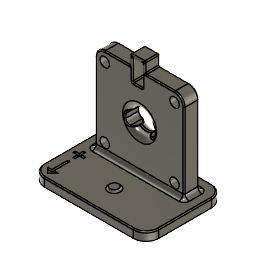
SOC Monitor Assembly (Autodesk Fusion 360 archive; units mm, degrees)
design "Mount"
part number: 2026-03-20-00-19-52-846
Autodesk Fusion 360 part; units mm, degrees
sketch "Base Bottom" plane through (0, 0, 0) normal (0, 0, 1) x (1, 0, 0)
  line L0 (-21, -18.5) -> (21, -18.5)
  line L1 (27, -12.5) -> (27, 12.5)
  line L2 (21, 18.5) -> (-21, 18.5)
  line L3 (-27, 12.5) -> (-27, -12.5)
  arc A0 (-21, 18.5) -> (-27, 12.5) centre (-21, 12.5) ccw
  arc A1 (-27, -12.5) -> (-21, -18.5) centre (-21, -12.5) ccw
  arc A2 (21, -18.5) -> (27, -12.5) centre (21, -12.5) ccw
  arc A3 (27, 12.5) -> (21, 18.5) centre (21, 12.5) ccw
  dimension "d125" = 6
  constraint tangent L2 A0
  constraint tangent L3 A0
  constraint tangent L3 A1
  constraint tangent L0 A1
  constraint equal A0 A1
  constraint tangent L0 A2
  constraint tangent L1 A2
  constraint equal A0 A2
  constraint tangent L1 A3
  constraint tangent L2 A3
  constraint equal A0 A3
  measures "d125" radius of A0
extrude "Extrude18" add sketch "Base Bottom" along normal blind 4
sketch "Base Top" plane through (0, 0, 4) normal (0, 0, 1) x (-1, 0, 0)
  arc A0 (-27, -12.5) -> (-21, -18.5) centre (-21, -12.5) ccw
  line L0 (-21, -18.5) -> (21, -18.5)
  arc A1 (21, -18.5) -> (27, -12.5) centre (21, -12.5) ccw
  line L1 (27, -12.5) -> (27, 12.5)
  arc A2 (27, 12.5) -> (21, 18.5) centre (21, 12.5) ccw
  line L2 (21, 18.5) -> (-21, 18.5)
  arc A3 (-21, 18.5) -> (-27, 12.5) centre (-21, 12.5) ccw
  line L3 (-27, 12.5) -> (-27, -12.5)
  line L4 (-21, -5.5) -> (21, -5.5)
  line L5 (21, -5.5) -> (21, -12.5)
  line L6 (21, -12.5) -> (-21, -12.5)
  line L7 (-21, -12.5) -> (-21, -5.5)
  circle A4 centre (0, 6.5) radius 2
  line L8 (21.5, 13.5) -> (22.5, 13.5)
  line L9 (22.5, 13.5) -> (22.5, 8.5)
  line L10 (22.5, 8.5) -> (21.5, 8.5)
  line L11 (21.5, 8.5) -> (21.5, 13.5)
  line L12 (21.5, 13.5) -> (22.5, 8.5) construction
  line L13 (22.5, 13.5) -> (21.5, 8.5) construction
  line L14 (22, 13.5) -> (19.5, 13.5)
  line L15 (19.5, 13.5) -> (22, 16)
  line L16 (22, 16) -> (24.5, 13.5)
  line L17 (24.5, 13.5) -> (22, 13.5)
  line L18 (21.5, 8.5) -> (22.5, 8.5)
  line L19 (22.5, 8.5) -> (22.5, 6)
  line L20 (22.5, 6) -> (21.5, 6)
  line L21 (21.5, 6) -> (21.5, 8.5)
  line L22 (22.5, -1.5) -> (21.5, -1.5)
  line L23 (21.5, 3.5) -> (22.5, 3.5)
  line L24 (21.5, 3.5) -> (21.5, -1.5)
  line L25 (22.5, -1.5) -> (22.5, 3.5)
  line L26 (19.5, 0.5) -> (24.5, 0.5)
  line L27 (24.5, 0.5) -> (24.5, 1.5)
  line L28 (24.5, 1.5) -> (19.5, 1.5)
  line L29 (19.5, 1.5) -> (19.5, 0.5)
  line L30 (19.5, 0.5) -> (24.5, 1.5) construction
  line L31 (24.5, 0.5) -> (19.5, 1.5) construction
  point P0 (22, 11)
  point P1 (22, 1)
  dimension "d135" = 42
  dimension "d136" = 7
  dimension "d195" = 4
  constraint horizontal L4
  constraint vertical L5
  constraint horizontal L6
  constraint vertical L7
  constraint horizontal L8
  constraint perpendicular L8 L9
  constraint parallel L8 L10
  constraint parallel L9 L11
  constraint coincident L12 P0
  constraint coincident L13 P0
  constraint midpoint L8 L14.start
  constraint parallel L8 L14
  constraint perpendicular L15 L16
  constraint parallel L8 L17
  constraint horizontal L18
  constraint vertical L19
  constraint horizontal L20
  constraint vertical L21
  constraint horizontal L23
  constraint perpendicular L22 L24
  constraint perpendicular L23 L25
  constraint horizontal L26
  constraint perpendicular L26 L27
  constraint parallel L26 L28
  constraint parallel L27 L29
  constraint coincident L30 P1
  constraint coincident L31 P1
  measures "d135" distance of L4.start L4.end
  measures "d136" distance of L4.start A0.centre
  measures "d195" diameter of A4
extrude "Extrude19" add sketch "Base Top" along normal blind 42 contours L4 L5 L6 L7
sketch "Mount" plane through (0, 5.5, 0) normal (0, -1, 0) x (1, 0, 0)
  line L0 (-21, 4) -> (21, 4)
  line L1 (21, 4) -> (21, 46)
  line L2 (21, 46) -> (-21, 46)
  line L3 (-21, 46) -> (-21, 4)
  line L4 (-21, 46) -> (21, 46)
  line L5 (21, 46) -> (21, 4)
  line L6 (21, 4) -> (-21, 4)
  line L7 (-21, 4) -> (-21, 46)
  circle A0 centre (0, 25) radius 20
  circle A1 centre (0, 25) radius 5
  line L8 (16.5, 41.5) -> (-16.5, 41.5)
  line L9 (-16.5, 41.5) -> (-16.5, 8.5)
  line L10 (-16.5, 8.5) -> (16.5, 8.5)
  line L11 (16.5, 8.5) -> (16.5, 41.5)
  circle A2 centre (16.5, 41.5) radius 2.25
  circle A3 centre (-16.5, 41.5) radius 2.25
  circle A4 centre (16.5, 8.5) radius 2.25
  circle A5 centre (-16.5, 8.5) radius 2.25
  line L12 (0, 35) -> (0, 51)
  line L13 (0, 51) -> (2, 51)
  line L14 (2.5, 51) -> (2.5, 39.62)
  line L15 (2.5, 39.62) -> (0, 39.62)
  line L16 (0, 39.62) -> (0, 51)
  line L17 (0, 51) -> (-4.5, 51)
  line L18 (-4.5, 51) -> (-4.5, 39.62)
  line L19 (-4.5, 39.62) -> (0, 39.62)
  line L20 (0, 39.62) -> (0, 51)
  line L21 (2.5, 51) -> (-4, 51)
  line L22 (-4.5, 50.5) -> (-4.5, 35)
  line L23 (-4.5, 35) -> (2.5, 35)
  line L24 (2.5, 35) -> (2.5, 50.5)
  line L25 (-3.5, 50) -> (-3.5, 36)
  line L26 (-3.5, 36) -> (1.5, 36)
  line L27 (1.5, 36) -> (1.5, 50)
  line L28 (1.5, 50) -> (-3.5, 50)
  arc A6 (2.5, 50.5) -> (2, 51) centre (2, 50.5) ccw
  arc A7 (-4, 51) -> (-4.5, 50.5) centre (-4, 50.5) ccw
  line L29 (7, 27) -> (-7, 27)
  line L30 (-7, 27) -> (-7, 21)
  line L31 (-7, 21) -> (7, 21)
  line L32 (7, 21) -> (7, 27)
  line L33 (7, 27) -> (-7, 21) construction
  line L34 (-7, 27) -> (7, 21) construction
  point P0 (0, 25)
  point P1 (-4.5, 51)
  point P2 (0, 24)
  dimension "d141" = 40
  dimension "d142" = 10
  dimension "d143" = 33
  dimension "d144" = 33
  dimension "d145" = 4.5
  dimension "d148" = -33
  dimension "d149" = -33
  dimension "d151" = 16
  dimension "d152" = 2.5
  dimension "d153" = 11.38
  dimension "d154" = 4.5
  dimension "d155" = 11.38
  dimension "d156" = 7
  dimension "d157" = 16
  dimension "d159" = 0.5
  constraint horizontal L4
  constraint vertical L5
  constraint horizontal L6
  constraint vertical L7
  constraint coincident L0.end L1.start
  constraint coincident L2.end L3.start
  constraint concentric A0 A1
  constraint horizontal L8
  constraint perpendicular L8 L9
  constraint parallel L8 L10
  constraint parallel L9 L11
  constraint coincident P0 A0.centre
  constraint coincident L8.start L11.end
  constraint perpendicular L8 L12
  constraint horizontal L13
  constraint vertical L14
  constraint horizontal L15
  constraint vertical L16
  constraint horizontal L17
  constraint vertical L18
  constraint horizontal L19
  constraint vertical L20
  constraint horizontal L21
  constraint vertical L22
  constraint horizontal L23
  constraint vertical L24
  constraint coincident L14.start L24
  constraint coincident L14.start L13
  constraint tangent L24 A6
  constraint tangent L13 A6
  constraint coincident P1 L21
  constraint coincident P1 L22
  constraint tangent L21 A7
  constraint tangent L22 A7
  constraint equal A6 A7
  constraint horizontal L29
  constraint perpendicular L29 L30
  constraint parallel L29 L31
  constraint parallel L30 L32
  constraint coincident L33 P2
  constraint coincident L34 P2
  measures "d141" diameter of A0
  measures "d142" diameter of A1
  measures "d143" distance of L9.end L10.end
  measures "d144" distance of L8.end L9.end
  measures "d145" diameter of A2
  measures "d151" distance of L12.start L12.end
  measures "d152" distance of L12.end L14.start
  measures "d153" distance of L12.end L15.end
  measures "d154" distance of L12.end P1
  measures "d155" distance of L12.end L15.end
  measures "d156" distance of L14.start P1
  measures "d157" distance of L14.start L23.end
  measures "d159" radius of A6
extrude "Extrude21" add sketch "Mount" against normal blind 7 contours L2 L4 L12 L16 L17 L18 L20 L21 L22 L25 L28 A7 | L2 L4 L12 L13 L14 L16 L20 L21 L24 L27 L28 A6
extrude "Extrude22" cut sketch "Mount" against normal blind 7 contours L2 L4 A0 L12 L16 L20 L25 | L2 L4 A0 L12 L16 L20 L27 | A0 L8 L12 L16 L20 L25 | A0 L8 L12 L16 L20 L27 | L8 L12 L16 L19 L20 L25 | L8 L12 L15 L16 L20 L27
fillet "Fillet18" radius 4.5 2 edges at (21, 9, 46) (-21, 9, 46)
extrude "Extrude23" cut sketch "Mount" against normal blind 6 contours L8 L9 A3 | L8 L9 A3 | L8 L11 A2 | L8 L11 A2 | L9 L10 A5 | L9 L10 A5 | L10 L11 A4 | L10 L11 A4
fillet "Fillet19" radius 0.5 22 edges at (9.5, 5.5, 46) (19.682, 5.5, 44.682) (21, 5.5, 22.75) (-21, 5.5, 22.75) (-19.682, 5.5, 44.682) (-10.5, 5.5, 46) (21, 12.5, 22.75) (19.682, 12.5, 44.682) (9.5, 12.5, 46) (-10.5, 12.5, 46) (-19.682, 12.5, 44.682) (-21, 12.5, 22.75) (2.5, 5.5, 48.25) (2.3536, 5.5, 50.8536) (-1, 5.5, 51) (-4.3536, 5.5, 50.8536) (-4.5, 5.5, 48.25) (-4.5, 12.5, 48.25) (-4.3536, 12.5, 50.8536) (-1, 12.5, 51) (2.3536, 12.5, 50.8536) (2.5, 12.5, 48.25)
fillet "Fillet20" radius 2 8 edges at (-20.8536, 5.6464, 4) (-21, 9, 4) (-20.8536, 12.3536, 4) (0, 12.5, 4) (20.8536, 12.3536, 4) (21, 9, 4) (20.8536, 5.6464, 4) (0, 5.5, 4)
fillet "Fillet22" radius 0.5 8 edges at (0, 18.5, 4) (-25.2426, 16.7426, 4) (-27, 0, 4) (-25.2426, -16.7426, 4) (0, -18.5, 4) (25.2426, -16.7426, 4) (27, 0, 4) (25.2426, 16.7426, 4)
extrude "Extrude24" cut sketch "Mount" against normal blind 7 contours A1 L29 L31 | A1 L29 | A1 L31
fillet "Fillet26" radius 0.5 4 edges at (1.5, 9, 39.62) (1.5, 9, 50) (-3.5, 9, 50) (-3.5, 9, 39.62)
fillet "Fillet27" radius 0.5 16 edges at (-3.3536, 5.5, 39.7664) (-3.5, 5.5, 44.81) (-3.3536, 5.5, 49.8536) (-1, 5.5, 50) (1.3536, 5.5, 49.8536) (1.5, 5.5, 44.81) (1.3536, 5.5, 39.7664) (-1, 5.5, 39.62) (1.3536, 12.5, 39.7664) (1.5, 12.5, 44.81) (1.3536, 12.5, 49.8536) (-1, 12.5, 50) (-3.3536, 12.5, 49.8536) (-3.5, 12.5, 44.81) (-3.3536, 12.5, 39.7664) (-1, 12.5, 39.62)
fillet "Fillet28" radius 3 2 edges at (-4.6616, 5.5, 26.8081) (-4.6616, 12.5, 23.1919)
fillet "Fillet30" radius 0.5 6 edges at (2.3536, 12.3536, 45.8536) (2.5, 9, 46) (2.3536, 5.6464, 45.8536) (-4.3536, 5.6464, 45.8536) (-4.5, 9, 46) (-4.3536, 12.3536, 45.8536)
extrude "Extrude25" add sketch "Base Top" along normal blind 0.9 contours A4
fillet "Fillet31" radius 0.9 1 edges at (1.8647, -7.2232, 4)
extrude "Extrude26" cut sketch "Mount" against normal blind 7 contours A1 L29 L31 L32 | A1 L29 L30 L31
fillet "Fillet32" radius 2 4 edges at (-7, 9, 21) (-7, 9, 27) (7, 9, 27) (7, 9, 21)
fillet "Fillet33" radius 0.5 24 edges at (3.6504, 6.9815, 21) (3, 9, 21) (3.6504, 11.0185, 21) (6.392, 12.4065, 21.5639) (7, 12.3534, 24.0172) (6.2667, 12.0716, 26.5477) (4.695, 10.2704, 27) (4.5826, 9, 27) (4.695, 7.7296, 27) (6.2758, 5.9241, 26.5402) (7, 5.6466, 24.0172) (6.3949, 5.5931, 21.5668) (-3.6504, 6.9815, 21) (-3, 9, 21) (-3.6504, 11.0185, 21) (-6.3949, 12.4069, 21.5668) (-7, 12.3534, 24.0172) (-6.2758, 12.0758, 26.5402) (-4.695, 10.2704, 27) (-4.5826, 9, 27) (-4.695, 7.7296, 27) (-6.2667, 5.9284, 26.5477) (-7, 5.6466, 24.0172) (-6.392, 5.5935, 21.5639)
extrude "Extrude27" cut sketch "Base Top" against normal blind 1 contours L8 L14 L15 L16 L17 | L8 L9 L10 L11 L14 L17 L18 | L10 L18 L19 L20 L21 | L22 L24 L25 L26 | L24 L25 L26 L28 | L23 L24 L25 L28
extrude "Extrude28" cut sketch "Base Top" against normal blind 1 contours L25 L26 L27 L28 | L24 L26 L28 L29
